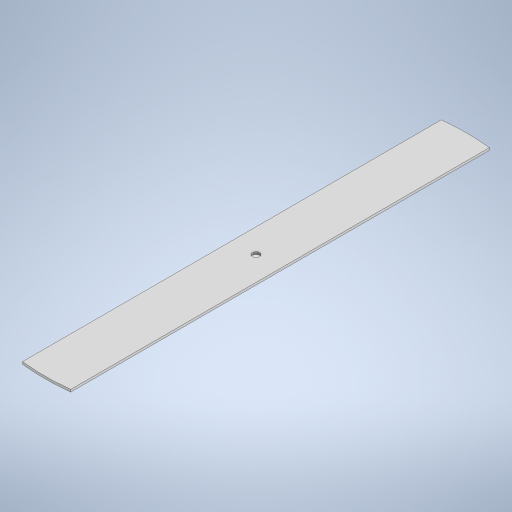
# Autodesk Inventor part: rotorV1
Saved by Autodesk Inventor 2024.4 (Build 284460000, 460)
## iProperties
Created: 2025-11-05
Part Number: rotorV1
Material: Generic
Document SubType Name: Modeling
Designer: jonas
Density: 1 g/cm^3
Appearance: Default
Author: jonas
Autodesk Inventor part; units mm, degrees
ref_plane "YZ Plane" through (0, 0, 0) normal (1, 0, 0) x (0, 1, 0)
ref_plane "XZ Plane" through (0, 0, 0) normal (0, 1, 0) x (-1, 0, 0)
ref_plane "XY Plane" through (0, 0, 0) normal (0, 0, 1) x (1, 0, 0)
sketch "Sketch1" plane through (0, 0, 0) normal (0, 1, 0) x (-1, 0, 0)
  line L0 (0, 272.2446) -> (0, -272.2446) construction
  line L1 (50, 435.2374) -> (50, -435.2374)
  line L2 (-50, 435.2374) -> (-50, -435.2374)
  arc A0 (50, 435.2374) -> (-50, 435.2374) centre (0, 0) ccw
  arc A1 (-50, -435.2374) -> (50, -435.2374) centre (0, 0) ccw
  circle A2 centre (0, 0) radius 7.5
  dimension "d1" = 438.1
  dimension "d2" = 438.1
  dimension "d3" = 100
  dimension "d6" = 15
  constraints: 6 end point, 4 point on circle, 3 centre point, 3 coincident, 3 vertical, 1 midpoint, 1 other
  measures "d1" radius of A1
  measures "d2" radius of A0
  measures "d3" distance between parallel lines of L2 L1
  measures "d6" diameter of A2
extrude "Extrusion1" add sketch "Sketch1" along normal blind 5
body "Solid1"
